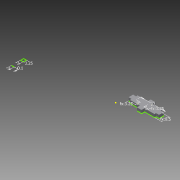
# Autodesk Inventor part: arm-servo
Saved by Autodesk Inventor 2013 (Build 170138000, 138)
## iProperties
Created: 2012-09-08
Part Number: arm-servo
Material: Generic
Document SubType Name: Modeling
Designer: frankenteddy
Density: 1 g/cm^3
Author: frankenteddy
Autodesk Inventor part; units mm, degrees
ref_plane "YZ Plane" through (0, 0, 0) normal (1, 0, 0) x (0, 1, 0)
ref_plane "XZ Plane" through (0, 0, 0) normal (0, 1, 0) x (-1, 0, 0)
ref_plane "XY Plane" through (0, 0, 0) normal (0, 0, 1) x (1, 0, 0)
sketch "Block1" plane through (0, 0, 0) normal (0, 0, 1) x (1, 0, 0)
  circle A0 centre (74.029, 24.2723) radius 1
  line L0 (49.279, 30.4723) -> (71.779, 30.4723)
  line L1 (71.779, 30.4723) -> (71.779, 18.0723)
  line L2 (71.779, 18.0723) -> (49.279, 18.0723)
  line L3 (49.279, 18.0723) -> (49.279, 30.4723)
  line L4 (49.279, 30.4723) -> (44.779, 30.4723)
  line L5 (44.779, 30.4723) -> (44.779, 18.0723)
  line L6 (44.779, 18.0723) -> (49.279, 18.0723)
  line L7 (49.279, 18.0723) -> (49.279, 30.4723)
  line L8 (71.779, 30.4723) -> (76.279, 30.4723)
  line L9 (76.279, 30.4723) -> (76.279, 18.0723)
  line L10 (76.279, 18.0723) -> (71.779, 18.0723)
  line L11 (71.779, 18.0723) -> (71.779, 30.4723)
  line L12 (44.779, 24.2723) -> (76.279, 24.2723) construction
  line L13 (47.029, 30.4723) -> (47.029, 18.0723) construction
  circle A1 centre (47.029, 24.2723) radius 1
  line L14 (74.029, 30.4723) -> (74.029, 18.0723) construction
  point P0 (60.979, 24.0984)
  dimension "d7" = 22.5
  dimension "d8" = 12.4
  dimension "d9" = 4.5
  dimension "d10" = 4.5
  dimension "d11" = 2
  dimension "d12" = 2
  measures "d7" distance of L1.end L2.end
  measures "d8" distance of L0.end L1.end
  measures "d9" distance of L6.end L5.end
  measures "d10" distance of L9.end L10.end
  measures "d11" diameter of A0
  measures "d12" diameter of A1
sketch "Sketch1" plane through (0, 0, 0) normal (0, 0, 1) x (1, 0, 0)
  line L0 (-92.7646, -8.503) -> (-89.7646, -8.503)
  line L1 (-89.7646, -8.503) -> (-89.7646, -11.753)
  line L2 (-89.7646, -11.753) -> (-92.7646, -11.753)
  line L3 (-92.7646, -11.753) -> (-92.7646, -8.503)
  line L4 (-92.7646, -21.6527) -> (-89.7646, -21.6527)
  line L5 (-89.7646, -21.6527) -> (-89.7646, -21.7527)
  line L6 (-89.7646, -21.7527) -> (-92.7646, -21.7527)
  line L7 (-92.7646, -21.7527) -> (-92.7646, -21.6527)
  line L8 (8.2668, 7.2563) -> (35.2668, 7.2563)
  line L9 (35.2668, 7.2563) -> (35.2668, 15.7563)
  line L10 (35.2668, 15.7563) -> (8.2668, 15.7563)
  line L11 (8.2668, 15.7563) -> (8.2668, 7.2563)
  line L12 (8.2668, 11.5063) -> (35.2668, 11.5063) construction
  line L13 (21.7668, 15.7563) -> (21.7668, 7.2563) construction
  line L14 (19.2668, 19.0063) -> (24.2668, 19.0063)
  line L15 (24.2668, 19.0063) -> (24.2668, 15.7563)
  line L16 (24.2668, 15.7563) -> (19.2668, 15.7563)
  line L17 (19.2668, 15.7563) -> (19.2668, 19.0063)
  line L18 (21.7668, 19.0063) -> (21.7668, 15.7563) construction
  line L19 (19.2668, 4.0063) -> (24.2668, 4.0063)
  line L20 (24.2668, 4.0063) -> (24.2668, 7.2563)
  line L21 (24.2668, 7.2563) -> (19.2668, 7.2563)
  line L22 (19.2668, 7.2563) -> (19.2668, 4.0063)
  line L23 (21.7668, 4.0063) -> (21.7668, 7.2563) construction
  line L24 (5.0168, 14.0063) -> (8.2668, 14.0063)
  line L25 (8.2668, 14.0063) -> (8.2668, 9.0063)
  line L26 (8.2668, 9.0063) -> (5.0168, 9.0063)
  line L27 (5.0168, 9.0063) -> (5.0168, 14.0063)
  line L28 (5.0168, 11.5063) -> (8.2668, 11.5063) construction
  line L29 (38.5168, 14.0063) -> (35.2668, 14.0063)
  line L30 (35.2668, 14.0063) -> (35.2668, 9.0063)
  line L31 (35.2668, 9.0063) -> (38.5168, 9.0063)
  line L32 (38.5168, 9.0063) -> (38.5168, 14.0063)
  line L33 (38.5168, 11.5063) -> (35.2668, 11.5063) construction
  point P0 (0, 0)
  point P1 (21.7668, 4.0063)
  dimension "d0" = 3
  dimension "mat" = 3.25
  dimension "d2" = 3
  dimension "d3" = 0.1
  dimension "d58" = 27
  dimension "d59" = 8.5
  dimension "d62" = 5
  dimension "d63" = 3.25
  dimension "d64" = 3.25
  dimension "d65" = 5
  constraints: 68 end point, 13 symmetric about line, 9 parallel, 8 midpoint, 5 perpendicular, 4 collinear, 4 horizontal
  measures "d0" distance of L1.end L3.start
  measures "mat" distance of L1.start L1.end
  measures "d2" distance of L5.end L7.start
  measures "d3" distance of L5.start L5.end
  measures "d58" distance of L10.end L9.end
  measures "d59" distance of L9.end L8.end
  measures "d62" distance of L15.end L16.end
  measures "d63" distance of L14.end L15.end
  measures "d64" distance of L25.end L26.end
  measures "d65" distance of L24.end L25.end
extrude "Extrusion5" add sketch "Sketch1" along normal blind 3.25 contours L11 L10 L9 L8
extrude "Extrusion6" cut sketch "Sketch1" along normal blind 3.25 contours L8 L20 L19 L22 | L26 L27 L24 L11 | L9 L29 L32 L31 | L17 L14 L15 L10
extrude "Extrusion7" add sketch "Sketch1" along normal blind 3.25 contours L26 L27 L24 L11 | L9 L29 L32 L31
extrude "Extrusion8" add sketch "Sketch1" along normal blind 3.25 contours L8 L20 L19 L22 | L17 L14 L15 L10
equation "\"d63\" = mat"
equation "\"d64\" = mat"
equation "\"d60\" = mat"
equation "\"d66\" = mat"
equation "\"d68\" = mat"
equation "\"d70\" = mat"
body "Solid4"
